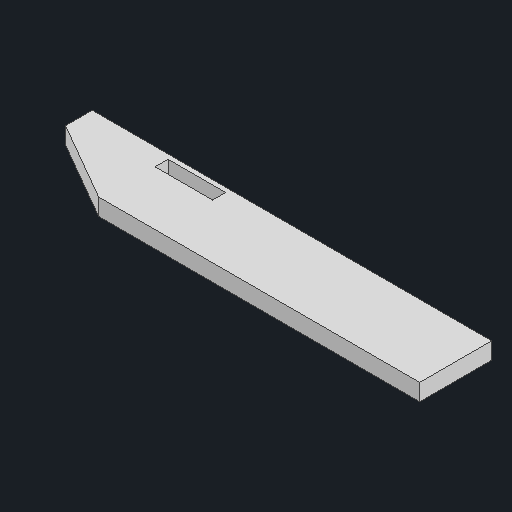
# Autodesk Inventor part: right_hold
Saved by Autodesk Inventor 2023 (Build 270158000, 158)
## iProperties
Created: 2024-04-29
Part Number: right_hold
Material: Generic
Document SubType Name: Modeling
Designer: szymo
Density: 1 g/cm^3
Appearance: Default
Mass: 35.07 g
Surface Area: 127.78 cm^2
Volume: 35.07 cm^3
Author: szymo
Autodesk Inventor part; units mm, degrees
ref_plane "YZ Plane" through (0, 0, 0) normal (1, 0, 0) x (0, 1, 0)
ref_plane "XZ Plane" through (0, 0, 0) normal (0, 1, 0) x (-1, 0, 0)
ref_plane "XY Plane" through (0, 0, 0) normal (0, 0, 1) x (1, 0, 0)
sketch "Sketch1" plane through (0, 0, 0) normal (0, 0, 1) x (1, 0, 0)
  line L0 (91, -34) -> (91, 34) projected
  line L1 (91, 34) -> (41, 34) projected
  line L2 (41, 34) -> (41, 89) projected
  line L3 (41, 89) -> (-91, 89) projected
  line L4 (-91, 89) -> (-91, -89) projected
  line L5 (-91, -89) -> (41, -89) projected
  line L6 (41, -89) -> (41, -34) projected
  line L7 (41, -34) -> (91, -34) projected
  line L8 (70, 27) -> (62, 27) projected
  line L9 (91, 34) -> (-87, 34)
  line L10 (-87, 34) -> (-87, 27)
  line L11 (-87, 27) -> (91, 27)
  line L12 (91, 27) -> (91, 34)
  circle A0 centre (-83, 21.5) radius 1.2295 projected
  circle A1 centre (-83, -64.5) radius 1.2295 projected
  circle A2 centre (-83, -21.5) radius 1.2295 projected
  circle A3 centre (-83, 64.5) radius 1.2295 projected
  line L13 (-85, -72) -> (-76, -72) projected
  line L14 (-76, -72) -> (-76, -57) projected
  line L15 (-76, -57) -> (-85, -57) projected
  arc A4 (-87, -55) -> (-85, -57) centre (-85, -55) ccw projected
  line L16 (-87, -55) -> (-87, -31) projected
  arc A5 (-85, -29) -> (-87, -31) centre (-85, -31) ccw projected
  line L17 (-85, -29) -> (-76, -29) projected
  line L18 (-76, -29) -> (-76, -14) projected
  line L19 (-76, -14) -> (-85, -14) projected
  arc A6 (-87, -12) -> (-85, -14) centre (-85, -12) ccw projected
  line L20 (-87, -12) -> (-87, 12) projected
  arc A7 (-85, 14) -> (-87, 12) centre (-85, 12) ccw projected
  line L21 (-85, 14) -> (-76, 14) projected
  line L22 (-76, 14) -> (-76, 29) projected
  line L23 (-76, 29) -> (-85, 29) projected
  arc A8 (-87, 31) -> (-85, 29) centre (-85, 31) ccw projected
  line L24 (-87, 31) -> (-87, 55) projected
  arc A9 (-85, 57) -> (-87, 55) centre (-85, 55) ccw projected
  line L25 (-85, 57) -> (-76, 57) projected
  line L26 (-76, 57) -> (-76, 72) projected
  line L27 (-76, 72) -> (-85, 72) projected
  arc A10 (-87, 74) -> (-85, 72) centre (-85, 74) ccw projected
  line L28 (-87, 74) -> (-87, 89) projected
  line L29 (-91, 89) -> (-87, 89) projected
  line L30 (-91, -89) -> (-91, 89) projected
  line L31 (-91, -89) -> (-87, -89) projected
  line L32 (-87, -89) -> (-87, -74) projected
  arc A11 (-85, -72) -> (-87, -74) centre (-85, -74) ccw projected
  line L33 (-91, 89.5) -> (-86.5, 89.5)
  line L34 (-86.5, 89.5) -> (-86.5, 74)
  arc A12 (-86.5, 74) -> (-85, 72.5) centre (-85, 74) ccw
  line L35 (-85, 72.5) -> (-75.5, 72.5)
  line L36 (-75.5, 72.5) -> (-75.5, 56.5)
  line L37 (-75.5, 56.5) -> (-85, 56.5)
  arc A13 (-85, 56.5) -> (-86.5, 55) centre (-85, 55) ccw
  line L38 (-86.5, 55) -> (-86.5, 31)
  arc A14 (-86.5, 31) -> (-85, 29.5) centre (-85, 31) ccw
  line L39 (-85, 29.5) -> (-75.5, 29.5)
  line L40 (-75.5, 29.5) -> (-75.5, 13.5)
  line L41 (-75.5, 13.5) -> (-85, 13.5)
  arc A15 (-85, 13.5) -> (-86.5, 12) centre (-85, 12) ccw
  line L42 (-86.5, 12) -> (-86.5, -12)
  arc A16 (-86.5, -12) -> (-85, -13.5) centre (-85, -12) ccw
  line L43 (-85, -13.5) -> (-75.5, -13.5)
  line L44 (-75.5, -13.5) -> (-75.5, -29.5)
  line L45 (-75.5, -29.5) -> (-85, -29.5)
  arc A17 (-85, -29.5) -> (-86.5, -31) centre (-85, -31) ccw
  line L46 (-86.5, -31) -> (-86.5, -55)
  arc A18 (-86.5, -55) -> (-85, -56.5) centre (-85, -55) ccw
  line L47 (-85, -56.5) -> (-75.5, -56.5)
  line L48 (-75.5, -56.5) -> (-75.5, -72.5)
  line L49 (-75.5, -72.5) -> (-85, -72.5)
  arc A19 (-85, -72.5) -> (-86.5, -74) centre (-85, -74) ccw
  line L50 (-86.5, -74) -> (-86.5, -89.5)
  line L51 (-86.5, -89.5) -> (-91, -89.5)
  line L52 (-86.5, 31) -> (-75.5, 31)
  line L53 (-75.5, 31) -> (-75.5, 29.5)
  line L54 (-75.5, 31) -> (-75.5, 34)
  point P0 (0, 0)
  point P1 (-75.5, 27)
  point P2 (-86.5, 34)
  dimension "d6" = 0.5
  constraints: 52 end point, 16 point on circle, 8 centre point, 3 perpendicular, 2 collinear, 2 horizontal, 2 parallel, 1 point on line, 26 other
  measures "d6" distance between parallel lines of L22 L40
extrude "Extrusion1" add sketch "Sketch1" along normal blind 30 contours L11 L8 L40 L53 L54 L9 L1 L0
sketch "Sketch3" plane through (-86.5, 34, 0) normal (0, 1, 0) x (1, 0, 0)
  line L0 (-0.5, -4.5) -> (-0.5, 0) projected
  line L1 (-0.5, 0) -> (-4.5, 0) projected
  line L2 (-4.5, 0) -> (-4.5, 3.5) projected
  line L3 (-4.5, 3.5) -> (-18.5, 3.5) projected
  line L4 (-18.5, 3.5) -> (-4.5, -5.5) projected
  line L5 (-4.5, -5.5) -> (-4.5, -4.5) projected
  line L6 (-4.5, -4.5) -> (-0.5, -4.5) projected
  line L7 (-0.5, -4.5) -> (50.0525, -33.6865)
  line L8 (177.5, 0) -> (11, 0) projected
  line L9 (177.5, -30) -> (11, -30) projected
  line L10 (177.5, 0) -> (177.5, -30) projected
  line L11 (11, 0) -> (11, -30) projected
  point P0 (86.5, 0)
  point P1 (43.6673, -30)
  point P2 (11, -11.1395)
  dimension "d7" = 30
  constraints: 2 end point
  measures "d7" angle of L7 L6
extrude "Extrusion4" cut sketch "Sketch3" against normal blind 30 contours L7 L9 L11
sketch "Sketch5" plane through (-75.5, 27, 0) normal (0, -1, 0) x (1, 0, 0)
  line L0 (56.5, 7.0341) -> (57.5, 7.0341) projected
  line L1 (34.5, 7.0341) -> (56.5, 7.0341) projected
  line L2 (33.5, 7.0341) -> (33.5, 6.6226)
  line L3 (33.5, 6.6226) -> (9.5, 6.6226)
  line L4 (9.5, 6.6226) -> (9.5, 7.0341)
  line L5 (9.5, 7.0341) -> (33.5, 7.0341)
  line L6 (64.5, 7.0341) -> (64.5, 6.6226)
  line L7 (64.5, 6.6226) -> (57.5, 6.6226)
  line L8 (57.5, 6.6226) -> (57.5, 7.0341)
  line L9 (57.5, 7.0341) -> (64.5, 7.0341)
  line L10 (9.5, 2) -> (9.5, 2.6226)
  line L11 (9.5, 2.6226) -> (64.5, 2.6226)
  line L12 (64.5, 2.6226) -> (64.5, 2)
  line L13 (64.5, 2) -> (9.5, 2)
  line L14 (9.5, 7.0341) -> (64.5, 7.0341)
  line L15 (64.5, 7.0341) -> (64.5, 2)
  line L16 (64.5, 2) -> (9.5, 2)
  line L17 (9.5, 2) -> (9.5, 7.0341)
  line L18 (9.2, 7.3341) -> (64.8, 7.3341)
  line L19 (64.8, 7.3341) -> (64.8, 1.9)
  line L20 (64.8, 1.9) -> (9.2, 1.9)
  line L21 (9.2, 1.9) -> (9.2, 7.3341)
  point P0 (75.5, 0)
  dimension "d19" = 0.3
  dimension "d20" = 0.3
  dimension "d21" = 0.1
  dimension "d22" = 0.3
  constraints: 40 end point, 8 horizontal, 6 vertical, 4 parallel, 2 perpendicular, 11 other
  measures "d19" distance between parallel lines of L21 L17
  measures "d20" distance between parallel lines of L19 L15
  measures "d21" distance between parallel lines of L13 L20
  measures "d22" distance between parallel lines of L18 L1
extrude "Extrusion6" cut sketch "Sketch5" against normal blind 0.7 contours L0 L8 L7 L15 L11 L17 L3 L2 L14 L1 | L9 L6 L7 L8 | L2 L3 L4 L5 | L12 L13 L10 L11 | L18 L19 L20 L21
sketch "Sketch6" plane through (-75.5, 27, 0) normal (0, -1, 0) x (1, 0, 0)
  line L0 (33.5, 7.0341) -> (34.5, 7.0341) projected
  line L1 (34.5, 7.0341) -> (56.5, 7.0341) projected
  line L2 (56.5, 7.0341) -> (57.5, 7.0341) projected
  line L3 (64.8, 1.9) -> (9.2, 1.9) projected
  line L4 (64.8, 7.3341) -> (64.8, 1.9) projected
  line L5 (9.2, 7.3341) -> (64.8, 7.3341) projected
  line L6 (9.2, 1.9) -> (9.2, 7.3341) projected
  line L7 (33.5, 7.3341) -> (57.5, 7.3341)
  line L8 (57.5, 7.3341) -> (57.5, 1.9)
  line L9 (57.5, 1.9) -> (33.5, 1.9)
  line L10 (33.5, 1.9) -> (33.5, 7.3341)
  point P0 (75.5, 0)
  constraints: 8 end point, 4 point on line, 2 parallel, 1 horizontal, 1 perpendicular
extrude "Extrusion7" cut sketch "Sketch6" against normal up to next contours L10 L5 L8 L2 L1 L0 | L0 L1 L2 L8 L3 L10
body "Solid1"
